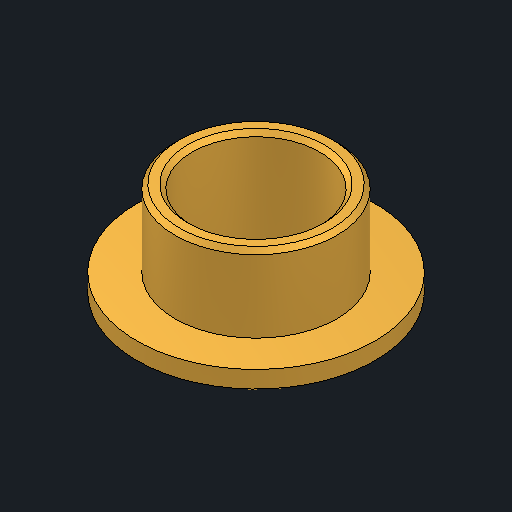
# Autodesk Inventor part: KN-00-02-06
Saved by Autodesk Inventor 2025.2 (Build 292293000, 293)
## iProperties
Created: 2025-04-13
Part Number: KN-00-02-06
Material: CuZn40
Document SubType Name: Modeling
Designer: Kacper Mik
Density: 8.47 g/cm^3
Appearance: Brass - Satin
Mass: 22.5272 g
Surface Area: 23.4862 cm^2
Volume: 2.65965 cm^3
Author: Kacper Mik
Autodesk Inventor part; units mm, degrees
ref_plane "YZ Plane" through (0, 0, 0) normal (1, 0, 0) x (0, 1, 0)
ref_plane "XZ Plane" through (0, 0, 0) normal (0, 1, 0) x (-1, 0, 0)
ref_plane "XY Plane" through (0, 0, 0) normal (0, 0, 1) x (1, 0, 0)
sketch "Sketch1" plane through (0, 0, 0) normal (0, 1, 0) x (-1, 0, 0)
  circle A0 centre (0, 0) radius 9.5
  dimension "d0" = 19
  constraints: 1 centre point, 1 coincident
  measures "d0" diameter of A0
extrude "Extrusion1" add sketch "Sketch1" along normal blind 9
sketch "Sketch2" plane through (0, 0, 0) normal (0, -1, 0) x (1, 0, 0)
  circle A0 centre (0, 0) radius 14
  dimension "d3" = 28
  constraints: 1 centre point, 1 coincident
  measures "d3" diameter of A0
extrude "Extrusion2" add sketch "Sketch2" along normal blind 2
sketch "Sketch5" plane through (0, 0, 0) normal (1, 0, 0) x (0, 1, 0)
  line L0 (-2, 14) -> (-2, -14) construction
  line L1 (-2, 0) -> (-2, 14)
  line L2 (-2, 0) -> (-7, 0)
  circle A0 centre (15.1, 0) radius 22.1 construction
  line L3 (-19.5566, 0) -> (77.1483, 0) projected
  arc A1 (-2, 14) -> (-7, 0) centre (15.1, 0) ccw
  point P0 (0, 0)
  dimension "d13" = 5
  constraints: 4 end point, 4 point on circle, 2 centre point, 1 collinear, 1 concentric, 1 midpoint, 1 perpendicular, 1 point on line
  measures "d13" distance of L1.start L2.end
revolve "Revolution1" add sketch "Sketch5" angle 360 about axis through (0, -10, 0) along (0, 1, 0)
sketch "Sketch6" plane through (0, 9, 0) normal (0, 1, 0) x (1, 0, 0)
  point P0 (0, 0)
  point P1 (0, 0)
  constraints: 1 coincident
hole "Hole2" at (0, 9, 0) direction (0, -1, 0) diameter 15 end through all
chamfer "Chamfer2" distance 0.5 angle 45 2 edges at (9.5, 9, 0) (0, 9, -7.5)
body "Solid1"
